Autodesk Fusion 360 part; units mm, degrees
(part 19 of 40)
  line L749 (-24.8392, 62.4581) -> (-24.83, 62.6207) construction
  line L750 (-24.83, 62.6207) -> (-24.8199, 62.7835) construction
  line L751 (-24.8199, 62.7835) -> (-24.8088, 62.9464) construction
  line L752 (-24.8088, 62.9464) -> (-24.7967, 63.1095) construction
  line L753 (-24.7967, 63.1095) -> (-24.7838, 63.2727) construction
  line L754 (-24.7838, 63.2727) -> (-24.77, 63.436) construction
  line L755 (-24.77, 63.436) -> (-24.7552, 63.5995) construction
  line L756 (-24.7552, 63.5995) -> (-24.7396, 63.7631) construction
  line L757 (-24.7396, 63.7631) -> (-24.723, 63.9268) construction
  line L758 (-24.723, 63.9268) -> (-24.7056, 64.0906) construction
  line L759 (-24.7056, 64.0906) -> (-24.6873, 64.2545) construction
  line L760 (-24.6873, 64.2545) -> (-24.6681, 64.4185) construction
  line L761 (-24.6681, 64.4185) -> (-24.648, 64.5826) construction
  line L762 (-24.648, 64.5826) -> (-24.6271, 64.7468) construction
  line L763 (-24.6271, 64.7468) -> (-24.6054, 64.9111) construction
  line L764 (-24.6054, 64.9111) -> (-24.5828, 65.0755) construction
  line L765 (-24.5828, 65.0755) -> (-24.5593, 65.24) construction
  line L766 (-24.5593, 65.24) -> (-24.535, 65.4046) construction
  line L767 (-24.535, 65.4046) -> (-24.5098, 65.5692) construction
  line L768 (-24.5098, 65.5692) -> (-24.4839, 65.734) construction
  line L769 (-24.4839, 65.734) -> (-24.4571, 65.8987) construction
  line L770 (-24.4571, 65.8987) -> (-24.4294, 66.0636) construction
  line L771 (-24.4294, 66.0636) -> (-24.401, 66.2285) construction
  line L772 (-24.401, 66.2285) -> (-24.3718, 66.3935) construction
  line L773 (-24.3718, 66.3935) -> (-24.3417, 66.5585) construction
  line L774 (-24.3417, 66.5585) -> (-24.3108, 66.7236) construction
  line L775 (-24.3108, 66.7236) -> (-24.2792, 66.8887) construction
  line L776 (-24.2792, 66.8887) -> (-24.2532, 67.0208) construction
  line L777 (-24.2532, 67.0208) -> (-24.2334, 67.1199) construction
  line L778 (-24.2334, 67.1199) -> (-24.22, 67.186) construction
  line L779 (-24.22, 67.186) -> (-24.2132, 67.2191) construction
  line L780 (-31.1115, -52.5103) -> (-31.1272, -52.5368) construction
  line L781 (-31.1272, -52.5368) -> (-31.1594, -52.5895) construction
  line L782 (-31.1594, -52.5895) -> (-31.2097, -52.6672) construction
  line L783 (-31.2097, -52.6672) -> (-31.2807, -52.7681) construction
  line L784 (-31.2807, -52.7681) -> (-31.3748, -52.8906) construction
  line L785 (-31.3748, -52.8906) -> (-31.4727, -53.0106) construction
  line L786 (-31.4727, -53.0106) -> (-31.5729, -53.1289) construction
  line L787 (-31.5729, -53.1289) -> (-31.6744, -53.2464) construction
  line L788 (-31.6744, -53.2464) -> (-31.7767, -53.3634) construction
  line L789 (-31.7767, -53.3634) -> (-31.88, -53.4797) construction
  line L790 (-31.88, -53.4797) -> (-31.9844, -53.5951) construction
  line L791 (-31.9844, -53.5951) -> (-32.0903, -53.7094) construction
  line L792 (-32.0903, -53.7094) -> (-32.1981, -53.8224) construction
  line L793 (-32.1981, -53.8224) -> (-32.3077, -53.934) construction
  line L794 (-32.3077, -53.934) -> (-32.419, -54.0444) construction
  line L795 (-32.419, -54.0444) -> (-32.5316, -54.1537) construction
  line L796 (-32.5316, -54.1537) -> (-32.6455, -54.2622) construction
  line L797 (-32.6455, -54.2622) -> (-32.7603, -54.3698) construction
  line L798 (-32.7603, -54.3698) -> (-32.876, -54.4767) construction
  line L799 (-32.876, -54.4767) -> (-32.9927, -54.5828) construction
  line L800 (-32.9927, -54.5828) -> (-33.1105, -54.6881) construction
  line L801 (-33.1105, -54.6881) -> (-33.2292, -54.7926) construction
  line L802 (-33.2292, -54.7926) -> (-33.3491, -54.8961) construction
  line L803 (-33.3491, -54.8961) -> (-33.47, -54.9988) construction
  line L804 (-33.47, -54.9988) -> (-33.5919, -55.1007) construction
  line L805 (-33.5919, -55.1007) -> (-33.7148, -55.2017) construction
  line L806 (-33.7148, -55.2017) -> (-33.8386, -55.302) construction
  line L807 (-33.8386, -55.302) -> (-33.9633, -55.4015) construction
  line L808 (-33.9633, -55.4015) -> (-34.0888, -55.5003) construction
  line L809 (-34.0888, -55.5003) -> (-34.2151, -55.5984) construction
  line L810 (-34.2151, -55.5984) -> (-34.3423, -55.6957) construction
  line L811 (-34.3423, -55.6957) -> (-34.4703, -55.7923) construction
  line L812 (-34.4703, -55.7923) -> (-34.5991, -55.8881) construction
  line L813 (-34.5991, -55.8881) -> (-34.7288, -55.9832) construction
  line L814 (-34.7288, -55.9832) -> (-34.8592, -56.0776) construction
  line L815 (-34.8592, -56.0776) -> (-34.9905, -56.1712) construction
  line L816 (-34.9905, -56.1712) -> (-35.1224, -56.2642) construction
  line L817 (-35.1224, -56.2642) -> (-35.2552, -56.3564) construction
  line L818 (-35.2552, -56.3564) -> (-35.3886, -56.448) construction
  line L819 (-35.3886, -56.448) -> (-35.5228, -56.5388) construction
  line L820 (-35.5228, -56.5388) -> (-35.6577, -56.629) construction
  line L821 (-35.6577, -56.629) -> (-35.7933, -56.7185) construction
  line L822 (-35.7933, -56.7185) -> (-35.9295, -56.8073) construction
  line L823 (-35.9295, -56.8073) -> (-36.0665, -56.8955) construction
  line L824 (-36.0665, -56.8955) -> (-36.2042, -56.9829) construction
  line L825 (-36.2042, -56.9829) -> (-36.3425, -57.0697) construction
  line L826 (-36.3425, -57.0697) -> (-36.4815, -57.1558) construction
  line L827 (-36.4815, -57.1558) -> (-36.6211, -57.2413) construction
  line L828 (-36.6211, -57.2413) -> (-36.7614, -57.3261) construction
  line L829 (-36.7614, -57.3261) -> (-36.9023, -57.4102) construction
  line L830 (-36.9023, -57.4102) -> (-37.0438, -57.4937) construction
  line L831 (-37.0438, -57.4937) -> (-37.186, -57.5765) construction
  line L832 (-37.186, -57.5765) -> (-37.3288, -57.6587) construction
  line L833 (-37.3288, -57.6587) -> (-37.4721, -57.7403) construction
  line L834 (-37.4721, -57.7403) -> (-37.6161, -57.8212) construction
  line L835 (-37.6161, -57.8212) -> (-37.7607, -57.9014) construction
  line L836 (-37.7607, -57.9014) -> (-37.9058, -57.981) construction
  line L837 (-37.9058, -57.981) -> (-38.0515, -58.06) construction
  line L838 (-38.0515, -58.06) -> (-38.1978, -58.1383) construction
  line L839 (-38.1978, -58.1383) -> (-38.3447, -58.216) construction
  line L840 (-38.3447, -58.216) -> (-38.4921, -58.2931) construction
  line L841 (-38.4921, -58.2931) -> (-38.6401, -58.3695) construction
  line L842 (-38.6401, -58.3695) -> (-38.7886, -58.4453) construction
  line L843 (-38.7886, -58.4453) -> (-38.9377, -58.5205) construction
  line L844 (-38.9377, -58.5205) -> (-39.0873, -58.595) construction
  line L845 (-39.0873, -58.595) -> (-39.2374, -58.669) construction
  line L846 (-39.2374, -58.669) -> (-39.3881, -58.7423) construction
  line L847 (-39.3881, -58.7423) -> (-39.5393, -58.8149) construction
  line L848 (-39.5393, -58.8149) -> (-39.6909, -58.887) construction
  line L849 (-39.6909, -58.887) -> (-39.8431, -58.9584) construction
  line L850 (-39.8431, -58.9584) -> (-39.9653, -59.0151) construction
  line L851 (-39.9653, -59.0151) -> (-40.0572, -59.0573) construction
  line L852 (-40.0572, -59.0573) -> (-40.1185, -59.0853) construction
  line L853 (-40.1185, -59.0853) -> (-40.1492, -59.0993) construction
  line L854 (-52.5103, 31.1115) -> (-52.5368, 31.1272) construction
  line L855 (-52.5368, 31.1272) -> (-52.5895, 31.1594) construction
  line L856 (-52.5895, 31.1594) -> (-52.6672, 31.2097) construction
  line L857 (-52.6672, 31.2097) -> (-52.7681, 31.2807) construction
  line L858 (-52.7681, 31.2807) -> (-52.8906, 31.3748) construction
  line L859 (-52.8906, 31.3748) -> (-53.0106, 31.4727) construction
  line L860 (-53.0106, 31.4727) -> (-53.1289, 31.5729) construction
  line L861 (-53.1289, 31.5729) -> (-53.2464, 31.6744) construction
  line L862 (-53.2464, 31.6744) -> (-53.3634, 31.7767) construction
  line L863 (-53.3634, 31.7767) -> (-53.4797, 31.88) construction
  line L864 (-53.4797, 31.88) -> (-53.5951, 31.9844) construction
  line L865 (-53.5951, 31.9844) -> (-53.7094, 32.0903) construction
  line L866 (-53.7094, 32.0903) -> (-53.8224, 32.1981) construction
  line L867 (-53.8224, 32.1981) -> (-53.934, 32.3077) construction
  line L868 (-53.934, 32.3077) -> (-54.0444, 32.419) construction
  line L869 (-54.0444, 32.419) -> (-54.1537, 32.5316) construction
  line L870 (-54.1537, 32.5316) -> (-54.2622, 32.6455) construction
  line L871 (-54.2622, 32.6455) -> (-54.3698, 32.7603) construction
  line L872 (-54.3698, 32.7603) -> (-54.4767, 32.876) construction
  line L873 (-54.4767, 32.876) -> (-54.5828, 32.9927) construction
  line L874 (-54.5828, 32.9927) -> (-54.6881, 33.1105) construction
  line L875 (-54.6881, 33.1105) -> (-54.7926, 33.2292) construction
  line L876 (-54.7926, 33.2292) -> (-54.8961, 33.3491) construction
  line L877 (-54.8961, 33.3491) -> (-54.9988, 33.47) construction
  line L878 (-54.9988, 33.47) -> (-55.1007, 33.5919) construction
  line L879 (-55.1007, 33.5919) -> (-55.2017, 33.7148) construction
  line L880 (-55.2017, 33.7148) -> (-55.302, 33.8386) construction
  line L881 (-55.302, 33.8386) -> (-55.4015, 33.9633) construction
  line L882 (-55.4015, 33.9633) -> (-55.5003, 34.0888) construction
  line L883 (-55.5003, 34.0888) -> (-55.5984, 34.2151) construction
  line L884 (-55.5984, 34.2151) -> (-55.6957, 34.3423) construction
  line L885 (-55.6957, 34.3423) -> (-55.7923, 34.4703) construction
  line L886 (-55.7923, 34.4703) -> (-55.8881, 34.5991) construction
  line L887 (-55.8881, 34.5991) -> (-55.9832, 34.7288) construction
  line L888 (-55.9832, 34.7288) -> (-56.0776, 34.8592) construction
  line L889 (-56.0776, 34.8592) -> (-56.1712, 34.9905) construction
  line L890 (-56.1712, 34.9905) -> (-56.2642, 35.1224) construction
  line L891 (-56.2642, 35.1224) -> (-56.3564, 35.2552) construction
  line L892 (-56.3564, 35.2552) -> (-56.448, 35.3886) construction
  line L893 (-56.448, 35.3886) -> (-56.5388, 35.5228) construction
  line L894 (-56.5388, 35.5228) -> (-56.629, 35.6577) construction
  line L895 (-56.629, 35.6577) -> (-56.7185, 35.7933) construction
  line L896 (-56.7185, 35.7933) -> (-56.8073, 35.9295) construction
  line L897 (-56.8073, 35.9295) -> (-56.8955, 36.0665) construction
  line L898 (-56.8955, 36.0665) -> (-56.9829, 36.2042) construction
  line L899 (-56.9829, 36.2042) -> (-57.0697, 36.3425) construction
  line L900 (-57.0697, 36.3425) -> (-57.1558, 36.4815) construction
  line L901 (-57.1558, 36.4815) -> (-57.2413, 36.6211) construction
  line L902 (-57.2413, 36.6211) -> (-57.3261, 36.7614) construction
  line L903 (-57.3261, 36.7614) -> (-57.4102, 36.9023) construction
  line L904 (-57.4102, 36.9023) -> (-57.4937, 37.0438) construction
  line L905 (-57.4937, 37.0438) -> (-57.5765, 37.186) construction
  line L906 (-57.5765, 37.186) -> (-57.6587, 37.3288) construction
  line L907 (-57.6587, 37.3288) -> (-57.7403, 37.4721) construction
  line L908 (-57.7403, 37.4721) -> (-57.8212, 37.6161) construction
  line L909 (-57.8212, 37.6161) -> (-57.9014, 37.7607) construction
  line L910 (-57.9014, 37.7607) -> (-57.981, 37.9058) construction
  line L911 (-57.981, 37.9058) -> (-58.06, 38.0515) construction
  line L912 (-58.06, 38.0515) -> (-58.1383, 38.1978) construction
  line L913 (-58.1383, 38.1978) -> (-58.216, 38.3447) construction
  line L914 (-58.216, 38.3447) -> (-58.2931, 38.4921) construction
  line L915 (-58.2931, 38.4921) -> (-58.3695, 38.6401) construction
  line L916 (-58.3695, 38.6401) -> (-58.4453, 38.7886) construction
  line L917 (-58.4453, 38.7886) -> (-58.5205, 38.9377) construction
  line L918 (-58.5205, 38.9377) -> (-58.595, 39.0873) construction
  line L919 (-58.595, 39.0873) -> (-58.669, 39.2374) construction
  line L920 (-58.669, 39.2374) -> (-58.7423, 39.3881) construction
  line L921 (-58.7423, 39.3881) -> (-58.8149, 39.5393) construction
  line L922 (-58.8149, 39.5393) -> (-58.887, 39.6909) construction
  line L923 (-58.887, 39.6909) -> (-58.9584, 39.8431) construction
  line L924 (-58.9584, 39.8431) -> (-59.0151, 39.9653) construction
  line L925 (-59.0151, 39.9653) -> (-59.0573, 40.0572) construction
  line L926 (-59.0573, 40.0572) -> (-59.0853, 40.1185) construction
  line L927 (-59.0853, 40.1185) -> (-59.0993, 40.1492) construction
  line L928 (5.6951, 60.7685) -> (5.6979, 60.7993) construction
  line L929 (5.6979, 60.7993) -> (5.7029, 60.8609) construction
  line L930 (5.7029, 60.8609) -> (5.7078, 60.9533) construction
  line L931 (5.7078, 60.9533) -> (5.7097, 61.0766) construction
  line L932 (5.7097, 61.0766) -> (5.7056, 61.231) construction
  line L933 (5.7056, 61.231) -> (5.6969, 61.3856) construction
  line L934 (5.6969, 61.3856) -> (5.6854, 61.5403) construction
  line L935 (5.6854, 61.5403) -> (5.6723, 61.695) construction
  line L936 (5.6723, 61.695) -> (5.6583, 61.8498) construction
  line L937 (5.6583, 61.8498) -> (5.6431, 62.0045) construction
  line L938 (5.6431, 62.0045) -> (5.6265, 62.1593) construction
  line L939 (5.6265, 62.1593) -> (5.608, 62.314) construction
  line L940 (5.608, 62.314) -> (5.5871, 62.4688) construction
  line L941 (5.5871, 62.4688) -> (5.5641, 62.6235) construction
  line L942 (5.5641, 62.6235) -> (5.539, 62.7782) construction
  line L943 (5.539, 62.7782) -> (5.5121, 62.9329) construction
  line L944 (5.5121, 62.9329) -> (5.4838, 63.0875) construction
  line L945 (5.4838, 63.0875) -> (5.4542, 63.2421) construction
  line L946 (5.4542, 63.2421) -> (5.4233, 63.3966) construction
  line L947 (5.4233, 63.3966) -> (5.3913, 63.5511) construction
  line L948 (5.3913, 63.5511) -> (5.3579, 63.7055) construction
  line L949 (5.3579, 63.7055) -> (5.3232, 63.8598) construction
  line L950 (5.3232, 63.8598) -> (5.2871, 64.014) construction
  line L951 (5.2871, 64.014) -> (5.2497, 64.1682) construction
  line L952 (5.2497, 64.1682) -> (5.2109, 64.3222) construction
  line L953 (5.2109, 64.3222) -> (5.1709, 64.4762) construction
  line L954 (5.1709, 64.4762) -> (5.1297, 64.6301) construction
  line L955 (5.1297, 64.6301) -> (5.0873, 64.7839) construction
  line L956 (5.0873, 64.7839) -> (5.0439, 64.9376) construction
  line L957 (5.0439, 64.9376) -> (4.9993, 65.0912) construction
  line L958 (4.9993, 65.0912) -> (4.9536, 65.2447) construction
  line L959 (4.9536, 65.2447) -> (4.9068, 65.398) construction
  line L960 (4.9068, 65.398) -> (4.8589, 65.5513) construction
  line L961 (4.8589, 65.5513) -> (4.8099, 65.7044) construction
  line L962 (4.8099, 65.7044) -> (4.7599, 65.8574) construction
  line L963 (4.7599, 65.8574) -> (4.7087, 66.0103) construction
  line L964 (4.7087, 66.0103) -> (4.6566, 66.1631) construction
  line L965 (4.6566, 66.1631) -> (4.6035, 66.3158) construction
  line L966 (4.6035, 66.3158) -> (4.5493, 66.4683) construction
  line L967 (4.5493, 66.4683) -> (4.4942, 66.6206) construction
  line L968 (4.4942, 66.6206) -> (4.438, 66.7729) construction
  line L969 (4.438, 66.7729) -> (4.381, 66.925) construction
  line L970 (4.381, 66.925) -> (4.3229, 67.077) construction
  line L971 (4.3229, 67.077) -> (4.2639, 67.2288) construction
  line L972 (4.2639, 67.2288) -> (4.2039, 67.3804) construction
  line L973 (4.2039, 67.3804) -> (4.143, 67.532) construction
  line L974 (4.143, 67.532) -> (4.0812, 67.6833) construction
  line L975 (4.0812, 67.6833) -> (4.0185, 67.8345) construction
  line L976 (4.0185, 67.8345) -> (3.9548, 67.9856) construction
  line L977 (3.9548, 67.9856) -> (3.8903, 68.1365) construction
  line L978 (3.8903, 68.1365) -> (3.8249, 68.2872) construction
  line L979 (3.8249, 68.2872) -> (3.7585, 68.4378) construction
  line L980 (3.7585, 68.4378) -> (3.6913, 68.5882) construction
  line L981 (3.6913, 68.5882) -> (3.6233, 68.7384) construction
  line L982 (3.6233, 68.7384) -> (3.5543, 68.8885) construction
  line L983 (3.5543, 68.8885) -> (3.4846, 69.0384) construction
  line L984 (3.4846, 69.0384) -> (3.4139, 69.1881) construction
  line L985 (3.4139, 69.1881) -> (3.3425, 69.3376) construction
  line L986 (3.3425, 69.3376) -> (3.2701, 69.487) construction
  line L987 (3.2701, 69.487) -> (3.197, 69.6362) construction
  line L988 (3.197, 69.6362) -> (3.123, 69.7852) construction
  line L989 (3.123, 69.7852) -> (3.0482, 69.934) construction
  line L990 (3.0482, 69.934) -> (2.9726, 70.0826) construction
  line L991 (2.9726, 70.0826) -> (2.8962, 70.2311) construction
  line L992 (2.8962, 70.2311) -> (2.819, 70.3793) construction
  line L993 (2.819, 70.3793) -> (2.741, 70.5274) construction
  line L994 (2.741, 70.5274) -> (2.6622, 70.6752) construction
  line L995 (2.6622, 70.6752) -> (2.5826, 70.8229) construction
  line L996 (2.5826, 70.8229) -> (2.5023, 70.9703) construction
  line L997 (2.5023, 70.9703) -> (2.4211, 71.1176) construction
  line L998 (2.4211, 71.1176) -> (2.3556, 71.2352) construction
  line L999 (2.3556, 71.2352) -> (2.3061, 71.3234) construction
  line L1000 (2.3061, 71.3234) -> (2.2729, 71.3821) construction
  line L1001 (2.2729, 71.3821) -> (2.2563, 71.4115) construction
  line L1002 (40.3263, 45.8153) -> (40.3467, 45.8385) construction
  line L1003 (40.3467, 45.8385) -> (40.3868, 45.8854) construction
  line L1004 (40.3868, 45.8854) -> (40.4451, 45.9573) construction
  line L1005 (40.4451, 45.9573) -> (40.5192, 46.056) construction
  line L1006 (40.5192, 46.056) -> (40.6066, 46.1833) construction
  line L1007 (40.6066, 46.1833) -> (40.6904, 46.3135) construction
  line L1008 (40.6904, 46.3135) -> (40.772, 46.4454) construction
  line L1009 (40.772, 46.4454) -> (40.8524, 46.5782) construction
  line L1010 (40.8524, 46.5782) -> (40.932, 46.7117) construction
  line L1011 (40.932, 46.7117) -> (41.0107, 46.8458) construction
  line L1012 (41.0107, 46.8458) -> (41.0883, 46.9807) construction
  line L1013 (41.0883, 46.9807) -> (41.1642, 47.1168) construction
  line L1014 (41.1642, 47.1168) -> (41.2383, 47.2543) construction
  line L1015 (41.2383, 47.2543) -> (41.3106, 47.393) construction
  line L1016 (41.3106, 47.393) -> (41.3813, 47.5329) construction
  line L1017 (41.3813, 47.5329) -> (41.4504, 47.6738) construction
  line L1018 (41.4504, 47.6738) -> (41.5184, 47.8156) construction
  line L1019 (41.5184, 47.8156) -> (41.5853, 47.9581) construction
  line L1020 (41.5853, 47.9581) -> (41.6512, 48.1012) construction
  line L1021 (41.6512, 48.1012) -> (41.716, 48.245) construction
  line L1022 (41.716, 48.245) -> (41.7798, 48.3895) construction
  line L1023 (41.7798, 48.3895) -> (41.8424, 48.5347) construction
  line L1024 (41.8424, 48.5347) -> (41.9039, 48.6807) construction
  line L1025 (41.9039, 48.6807) -> (41.9642, 48.8274) construction
  line L1026 (41.9642, 48.8274) -> (42.0234, 48.9749) construction
  line L1027 (42.0234, 48.9749) -> (42.0815, 49.123) construction
  line L1028 (42.0815, 49.123) -> (42.1386, 49.2717) construction
  line L1029 (42.1386, 49.2717) -> (42.1947, 49.421) construction
  line L1030 (42.1947, 49.421) -> (42.2499, 49.5709) construction
  line L1031 (42.2499, 49.5709) -> (42.3041, 49.7214) construction
  line L1032 (42.3041, 49.7214) -> (42.3574, 49.8724) construction
  line L1033 (42.3574, 49.8724) -> (42.4097, 50.024) construction
  line L1034 (42.4097, 50.024) -> (42.461, 50.1761) construction
  line L1035 (42.461, 50.1761) -> (42.5114, 50.3288) construction
  line L1036 (42.5114, 50.3288) -> (42.5608, 50.482) construction
  line L1037 (42.5608, 50.482) -> (42.6094, 50.6358) construction
  line L1038 (42.6094, 50.6358) -> (42.657, 50.79) construction
  line L1039 (42.657, 50.79) -> (42.7037, 50.9447) construction
  line L1040 (42.7037, 50.9447) -> (42.7495, 51.0999) construction
  line L1041 (42.7495, 51.0999) -> (42.7945, 51.2556) construction
  line L1042 (42.7945, 51.2556) -> (42.8386, 51.4118) construction
  line L1043 (42.8386, 51.4118) -> (42.8818, 51.5684) construction
  line L1044 (42.8818, 51.5684) -> (42.9241, 51.7255) construction
  line L1045 (42.9241, 51.7255) -> (42.9656, 51.883) construction
  line L1046 (42.9656, 51.883) -> (43.0063, 52.0409) construction
  line L1047 (43.0063, 52.0409) -> (43.0461, 52.1993) construction
  line L1048 (43.0461, 52.1993) -> (43.085, 52.3581) construction
  line L1049 (43.085, 52.3581) -> (43.1231, 52.5173) construction
  line L1050 (43.1231, 52.5173) -> (43.1604, 52.6769) construction
  line L1051 (43.1604, 52.6769) -> (43.1969, 52.8369) construction
  line L1052 (43.1969, 52.8369) -> (43.2326, 52.9973) construction
  line L1053 (43.2326, 52.9973) -> (43.2674, 53.1581) construction
  line L1054 (43.2674, 53.1581) -> (43.3015, 53.3193) construction
  line L1055 (43.3015, 53.3193) -> (43.3347, 53.4809) construction
  line L1056 (43.3347, 53.4809) -> (43.3672, 53.6428) construction
  line L1057 (43.3672, 53.6428) -> (43.3988, 53.8051) construction
  line L1058 (43.3988, 53.8051) -> (43.4297, 53.9677) construction
  line L1059 (43.4297, 53.9677) -> (43.4597, 54.1307) construction
  line L1060 (43.4597, 54.1307) -> (43.489, 54.294) construction
  line L1061 (43.489, 54.294) -> (43.5175, 54.4577) construction
  line L1062 (43.5175, 54.4577) -> (43.5453, 54.6217) construction
  line L1063 (43.5453, 54.6217) -> (43.5723, 54.7861) construction
  line L1064 (43.5723, 54.7861) -> (43.5984, 54.9508) construction
  line L1065 (43.5984, 54.9508) -> (43.6239, 55.1158) construction
  line L1066 (43.6239, 55.1158) -> (43.6486, 55.2811) construction
  line L1067 (43.6486, 55.2811) -> (43.6725, 55.4467) construction
  line L1068 (43.6725, 55.4467) -> (43.6956, 55.6126) construction
  line L1069 (43.6956, 55.6126) -> (43.718, 55.7789) construction
  line L1070 (43.718, 55.7789) -> (43.7397, 55.9454) construction
  line L1071 (43.7397, 55.9454) -> (43.7606, 56.1122) construction
  line L1072 (43.7606, 56.1122) -> (43.7767, 56.2459) construction
  line L1073 (43.7767, 56.2459) -> (43.7885, 56.3463) construction
  line L1074 (43.7885, 56.3463) -> (43.7962, 56.4133) construction
  line L1075 (43.7962, 56.4133) -> (43.8, 56.4469) construction
  line L1076 (-59.5542, -13.3622) -> (-59.5843, -13.369) construction
  line L1077 (-59.5843, -13.369) -> (-59.6444, -13.3833) construction
  line L1078 (-59.6444, -13.3833) -> (-59.7338, -13.4071) construction
  line L1079 (-59.7338, -13.4071) -> (-59.8517, -13.4435) construction
  line L1080 (-59.8517, -13.4435) -> (-59.9973, -13.4951) construction
  line L1081 (-59.9973, -13.4951) -> (-60.1416, -13.5511) construction
  line L1082 (-60.1416, -13.5511) -> (-60.2852, -13.6099) construction
  line L1083 (-60.2852, -13.6099) -> (-60.4283, -13.6701) construction
  line L1084 (-60.4283, -13.6701) -> (-60.5711, -13.7313) construction
  line L1085 (-60.5711, -13.7313) -> (-60.7136, -13.7935) construction
  line L1086 (-60.7136, -13.7935) -> (-60.8557, -13.8571) construction
  line L1087 (-60.8557, -13.8571) -> (-60.9971, -13.9226) construction
  line L1088 (-60.9971, -13.9226) -> (-61.1379, -13.9902) construction
  line L1089 (-61.1379, -13.9902) -> (-61.2779, -14.06) construction
  line L1090 (-61.2779, -14.06) -> (-61.4173, -14.1316) construction
  line L1091 (-61.4173, -14.1316) -> (-61.5561, -14.205) construction
  line L1092 (-61.5561, -14.205) -> (-61.6944, -14.2797) construction
  line L1093 (-61.6944, -14.2797) -> (-61.8322, -14.3557) construction
  line L1094 (-61.8322, -14.3557) -> (-61.9697, -14.4327) construction
  line L1095 (-61.9697, -14.4327) -> (-62.1067, -14.5109) construction
  line L1096 (-62.1067, -14.5109) -> (-62.2432, -14.5904) construction
  line L1097 (-62.2432, -14.5904) -> (-62.3792, -14.6711) construction
  line L1098 (-62.3792, -14.6711) -> (-62.5148, -14.753) construction
  line L1099 (-62.5148, -14.753) -> (-62.6498, -14.8363) construction
  line L1100 (-62.6498, -14.8363) -> (-62.7843, -14.9208) construction
  line L1101 (-62.7843, -14.9208) -> (-62.9184, -15.0064) construction
  line L1102 (-62.9184, -15.0064) -> (-63.052, -15.0932) construction
  line L1103 (-63.052, -15.0932) -> (-63.1852, -15.181) construction
  line L1104 (-63.1852, -15.181) -> (-63.318, -15.2698) construction
  line L1105 (-63.318, -15.2698) -> (-63.4503, -15.3597) construction
  line L1106 (-63.4503, -15.3597) -> (-63.5821, -15.4506) construction
  line L1107 (-63.5821, -15.4506) -> (-63.7135, -15.5425) construction
  line L1108 (-63.7135, -15.5425) -> (-63.8445, -15.6354) construction
  line L1109 (-63.8445, -15.6354) -> (-63.975, -15.7293) construction
  line L1110 (-63.975, -15.7293) -> (-64.105, -15.8242) construction
  line L1111 (-64.105, -15.8242) -> (-64.2346, -15.92) construction
  line L1112 (-64.2346, -15.92) -> (-64.3638, -16.0168) construction
  line L1113 (-64.3638, -16.0168) -> (-64.4926, -16.1146) construction
  line L1114 (-64.4926, -16.1146) -> (-64.6209, -16.2132) construction
  line L1115 (-64.6209, -16.2132) -> (-64.7488, -16.3127) construction
  line L1116 (-64.7488, -16.3127) -> (-64.8762, -16.4131) construction
  line L1117 (-64.8762, -16.4131) -> (-65.0032, -16.5144) construction
  line L1118 (-65.0032, -16.5144) -> (-65.1298, -16.6166) construction
  line L1119 (-65.1298, -16.6166) -> (-65.256, -16.7196) construction
  line L1120 (-65.256, -16.7196) -> (-65.3817, -16.8235) construction
  line L1121 (-65.3817, -16.8235) -> (-65.507, -16.9283) construction
  line L1122 (-65.507, -16.9283) -> (-65.6318, -17.0338) construction
  line L1123 (-65.6318, -17.0338) -> (-65.7562, -17.1402) construction
  line L1124 (-65.7562, -17.1402) -> (-65.8802, -17.2474) construction
  line L1125 (-65.8802, -17.2474) -> (-66.0038, -17.3555) construction
  line L1126 (-66.0038, -17.3555) -> (-66.1269, -17.4643) construction
  line L1127 (-66.1269, -17.4643) -> (-66.2497, -17.5739) construction
  line L1128 (-66.2497, -17.5739) -> (-66.3719, -17.6842) construction
  line L1129 (-66.3719, -17.6842) -> (-66.4938, -17.7954) construction
  line L1130 (-66.4938, -17.7954) -> (-66.6152, -17.9073) construction
  line L1131 (-66.6152, -17.9073) -> (-66.7362, -18.02) construction
  line L1132 (-66.7362, -18.02) -> (-66.8568, -18.1335) construction
  line L1133 (-66.8568, -18.1335) -> (-66.9769, -18.2477) construction
  line L1134 (-66.9769, -18.2477) -> (-67.0966, -18.3626) construction
  line L1135 (-67.0966, -18.3626) -> (-67.2159, -18.4782) construction
  line L1136 (-67.2159, -18.4782) -> (-67.3347, -18.5946) construction
  line L1137 (-67.3347, -18.5946) -> (-67.4531, -18.7118) construction
  line L1138 (-67.4531, -18.7118) -> (-67.5711, -18.8296) construction
  line L1139 (-67.5711, -18.8296) -> (-67.6887, -18.9481) construction
  line L1140 (-67.6887, -18.9481) -> (-67.8058, -19.0674) construction
  line L1141 (-67.8058, -19.0674) -> (-67.9225, -19.1873) construction
  line L1142 (-67.9225, -19.1873) -> (-68.0388, -19.3079) construction
  line L1143 (-68.0388, -19.3079) -> (-68.1546, -19.4293) construction
  line L1144 (-68.1546, -19.4293) -> (-68.27, -19.5512) construction
  line L1145 (-68.27, -19.5512) -> (-68.385, -19.6739) construction
  line L1146 (-68.385, -19.6739) -> (-68.4767, -19.7726) construction
  line L1147 (-68.4767, -19.7726) -> (-68.5452, -19.8469) construction
  line L1148 (-68.5452, -19.8469) -> (-68.5908, -19.8966) construction
  line L1149 (-68.5908, -19.8966) -> (-68.6136, -19.9215) construction
  line L1150 (-52.5103, -31.1115) -> (-52.5368, -31.1272) construction
  line L1151 (-52.5368, -31.1272) -> (-52.5895, -31.1594) construction
  line L1152 (-52.5895, -31.1594) -> (-52.6672, -31.2097) construction
  line L1153 (-52.6672, -31.2097) -> (-52.7681, -31.2807) construction
  line L1154 (-52.7681, -31.2807) -> (-52.8906, -31.3748) construction
  line L1155 (-52.8906, -31.3748) -> (-53.0106, -31.4727) construction
  line L1156 (-53.0106, -31.4727) -> (-53.1289, -31.5729) construction
  line L1157 (-53.1289, -31.5729) -> (-53.2464, -31.6744) construction
  line L1158 (-53.2464, -31.6744) -> (-53.3634, -31.7767) construction
  line L1159 (-53.3634, -31.7767) -> (-53.4797, -31.88) construction
  line L1160 (-53.4797, -31.88) -> (-53.5951, -31.9844) construction
  line L1161 (-53.5951, -31.9844) -> (-53.7094, -32.0903) construction
  line L1162 (-53.7094, -32.0903) -> (-53.8224, -32.1981) construction
  line L1163 (-53.8224, -32.1981) -> (-53.934, -32.3077) construction
  line L1164 (-53.934, -32.3077) -> (-54.0444, -32.419) construction
  line L1165 (-54.0444, -32.419) -> (-54.1537, -32.5316) construction
  line L1166 (-54.1537, -32.5316) -> (-54.2622, -32.6455) construction
  line L1167 (-54.2622, -32.6455) -> (-54.3698, -32.7603) construction
  line L1168 (-54.3698, -32.7603) -> (-54.4767, -32.876) construction
  line L1169 (-54.4767, -32.876) -> (-54.5828, -32.9927) construction
  line L1170 (-54.5828, -32.9927) -> (-54.6881, -33.1105) construction
  line L1171 (-54.6881, -33.1105) -> (-54.7926, -33.2292) construction
  line L1172 (-54.7926, -33.2292) -> (-54.8961, -33.3491) construction
  line L1173 (-54.8961, -33.3491) -> (-54.9988, -33.47) construction
  line L1174 (-54.9988, -33.47) -> (-55.1007, -33.5919) construction
  line L1175 (-55.1007, -33.5919) -> (-55.2017, -33.7148) construction
  line L1176 (-55.2017, -33.7148) -> (-55.302, -33.8386) construction
  line L1177 (-55.302, -33.8386) -> (-55.4015, -33.9633) construction
  line L1178 (-55.4015, -33.9633) -> (-55.5003, -34.0888) construction
  line L1179 (-55.5003, -34.0888) -> (-55.5984, -34.2151) construction
  line L1180 (-55.5984, -34.2151) -> (-55.6957, -34.3423) construction
  line L1181 (-55.6957, -34.3423) -> (-55.7923, -34.4703) construction
  line L1182 (-55.7923, -34.4703) -> (-55.8881, -34.5991) construction
  line L1183 (-55.8881, -34.5991) -> (-55.9832, -34.7288) construction
  line L1184 (-55.9832, -34.7288) -> (-56.0776, -34.8592) construction
  line L1185 (-56.0776, -34.8592) -> (-56.1712, -34.9905) construction
  line L1186 (-56.1712, -34.9905) -> (-56.2642, -35.1224) construction
  line L1187 (-56.2642, -35.1224) -> (-56.3564, -35.2552) construction
  line L1188 (-56.3564, -35.2552) -> (-56.448, -35.3886) construction
  line L1189 (-56.448, -35.3886) -> (-56.5388, -35.5228) construction
  line L1190 (-56.5388, -35.5228) -> (-56.629, -35.6577) construction
  line L1191 (-56.629, -35.6577) -> (-56.7185, -35.7933) construction
  line L1192 (-56.7185, -35.7933) -> (-56.8073, -35.9295) construction
  line L1193 (-56.8073, -35.9295) -> (-56.8955, -36.0665) construction
  line L1194 (-56.8955, -36.0665) -> (-56.9829, -36.2042) construction
  line L1195 (-56.9829, -36.2042) -> (-57.0697, -36.3425) construction
  line L1196 (-57.0697, -36.3425) -> (-57.1558, -36.4815) construction
  line L1197 (-57.1558, -36.4815) -> (-57.2413, -36.6211) construction
  line L1198 (-57.2413, -36.6211) -> (-57.3261, -36.7614) construction
  line L1199 (-57.3261, -36.7614) -> (-57.4102, -36.9023) construction
  line L1200 (-57.4102, -36.9023) -> (-57.4937, -37.0438) construction
  line L1201 (-57.4937, -37.0438) -> (-57.5765, -37.186) construction
  line L1202 (-57.5765, -37.186) -> (-57.6587, -37.3288) construction
  line L1203 (-57.6587, -37.3288) -> (-57.7403, -37.4721) construction
  line L1204 (-57.7403, -37.4721) -> (-57.8212, -37.6161) construction
  line L1205 (-57.8212, -37.6161) -> (-57.9014, -37.7607) construction
  line L1206 (-57.9014, -37.7607) -> (-57.981, -37.9058) construction
  line L1207 (-57.981, -37.9058) -> (-58.06, -38.0515) construction
  line L1208 (-58.06, -38.0515) -> (-58.1383, -38.1978) construction
  line L1209 (-58.1383, -38.1978) -> (-58.216, -38.3447) construction
  line L1210 (-58.216, -38.3447) -> (-58.2931, -38.4921) construction
  line L1211 (-58.2931, -38.4921) -> (-58.3695, -38.6401) construction
  line L1212 (-58.3695, -38.6401) -> (-58.4453, -38.7886) construction
  line L1213 (-58.4453, -38.7886) -> (-58.5205, -38.9377) construction
  line L1214 (-58.5205, -38.9377) -> (-58.595, -39.0873) construction
  line L1215 (-58.595, -39.0873) -> (-58.669, -39.2374) construction
  line L1216 (-58.669, -39.2374) -> (-58.7423, -39.3881) construction
  line L1217 (-58.7423, -39.3881) -> (-58.8149, -39.5393) construction
  line L1218 (-58.8149, -39.5393) -> (-58.887, -39.6909) construction
  line L1219 (-58.887, -39.6909) -> (-58.9584, -39.8431) construction
  line L1220 (-58.9584, -39.8431) -> (-59.0151, -39.9653) construction
  line L1221 (-59.0151, -39.9653) -> (-59.0573, -40.0572) construction
  line L1222 (-59.0573, -40.0572) -> (-59.0853, -40.1185) construction
  line L1223 (-59.0853, -40.1185) -> (-59.0993, -40.1492) construction
  line L1224 (-56.0345, -24.1948) -> (-56.0628, -24.2071) construction
  line L1225 (-56.0628, -24.2071) -> (-56.1198, -24.2308) construction
  line L1226 (-56.1198, -24.2308) -> (-56.2062, -24.264) construction
  line L1227 (-56.2062, -24.264) -> (-56.3229, -24.3039) construction
  line L1228 (-56.3229, -24.3039) -> (-56.4711, -24.3478) construction
  line L1229 (-56.4711, -24.3478) -> (-56.6208, -24.3873) construction
  line L1230 (-56.6208, -24.3873) -> (-56.7714, -24.4241) construction
  line L1231 (-56.7714, -24.4241) -> (-56.9226, -24.4595) construction
  line L1232 (-56.9226, -24.4595) -> (-57.0741, -24.494) construction
  line L1233 (-57.0741, -24.494) -> (-57.226, -24.5274) construction
  line L1234 (-57.226, -24.5274) -> (-57.3783, -24.5594) construction
  line L1235 (-57.3783, -24.5594) -> (-57.5312, -24.5896) construction
  line L1236 (-57.5312, -24.5896) -> (-57.6848, -24.6176) construction
  line L1237 (-57.6848, -24.6176) -> (-57.8391, -24.6435) construction
  line L1238 (-57.8391, -24.6435) -> (-57.994, -24.6674) construction
  line L1239 (-57.994, -24.6674) -> (-58.1494, -24.6897) construction
  line L1240 (-58.1494, -24.6897) -> (-58.3052, -24.7105) construction
  line L1241 (-58.3052, -24.7105) -> (-58.4614, -24.7301) construction
  line L1242 (-58.4614, -24.7301) -> (-58.6179, -24.7485) construction
  line L1243 (-58.6179, -24.7485) -> (-58.7747, -24.7658) construction
  line L1244 (-58.7747, -24.7658) -> (-58.9318, -24.7818) construction
  line L1245 (-58.9318, -24.7818) -> (-59.0893, -24.7965) construction
  line L1246 (-59.0893, -24.7965) -> (-59.2471, -24.8098) construction
  line L1247 (-59.2471, -24.8098) -> (-59.4053, -24.8218) construction
  line L1248 (-59.4053, -24.8218) -> (-59.5638, -24.8325) construction
  line L1249 (-59.5638, -24.8325) -> (-59.7226, -24.842) construction
  line L1250 (-59.7226, -24.842) -> (-59.8817, -24.8504) construction
  line L1251 (-59.8817, -24.8504) -> (-60.0411, -24.8577) construction
  line L1252 (-60.0411, -24.8577) -> (-60.2007, -24.8638) construction
  line L1253 (-60.2007, -24.8638) -> (-60.3605, -24.8689) construction
  line L1254 (-60.3605, -24.8689) -> (-60.5206, -24.8729) construction
  line L1255 (-60.5206, -24.8729) -> (-60.6809, -24.8757) construction
  line L1256 (-60.6809, -24.8757) -> (-60.8415, -24.8776) construction
  line L1257 (-60.8415, -24.8776) -> (-61.0023, -24.8783) construction
  line L1258 (-61.0023, -24.8783) -> (-61.1633, -24.878) construction
  line L1259 (-61.1633, -24.878) -> (-61.3245, -24.8766) construction
  line L1260 (-61.3245, -24.8766) -> (-61.4859, -24.8742) construction
  line L1261 (-61.4859, -24.8742) -> (-61.6475, -24.8708) construction
  line L1262 (-61.6475, -24.8708) -> (-61.8093, -24.8665) construction
  line L1263 (-61.8093, -24.8665) -> (-61.9712, -24.8611) construction
  line L1264 (-61.9712, -24.8611) -> (-62.1334, -24.8548) construction
  line L1265 (-62.1334, -24.8548) -> (-62.2957, -24.8475) construction
  line L1266 (-62.2957, -24.8475) -> (-62.4581, -24.8392) construction
  line L1267 (-62.4581, -24.8392) -> (-62.6207, -24.83) construction
  line L1268 (-62.6207, -24.83) -> (-62.7835, -24.8199) construction
  line L1269 (-62.7835, -24.8199) -> (-62.9464, -24.8088) construction
  line L1270 (-62.9464, -24.8088) -> (-63.1095, -24.7967) construction
  line L1271 (-63.1095, -24.7967) -> (-63.2727, -24.7838) construction
  line L1272 (-63.2727, -24.7838) -> (-63.436, -24.77) construction
  line L1273 (-63.436, -24.77) -> (-63.5995, -24.7552) construction
  line L1274 (-63.5995, -24.7552) -> (-63.7631, -24.7396) construction
  line L1275 (-63.7631, -24.7396) -> (-63.9268, -24.723) construction
  line L1276 (-63.9268, -24.723) -> (-64.0906, -24.7056) construction
  line L1277 (-64.0906, -24.7056) -> (-64.2545, -24.6873) construction
  line L1278 (-64.2545, -24.6873) -> (-64.4185, -24.6681) construction
  line L1279 (-64.4185, -24.6681) -> (-64.5826, -24.648) construction
  line L1280 (-64.5826, -24.648) -> (-64.7468, -24.6271) construction
  line L1281 (-64.7468, -24.6271) -> (-64.9111, -24.6054) construction
  line L1282 (-64.9111, -24.6054) -> (-65.0755, -24.5828) construction
  line L1283 (-65.0755, -24.5828) -> (-65.24, -24.5593) construction
  line L1284 (-65.24, -24.5593) -> (-65.4046, -24.535) construction
  line L1285 (-65.4046, -24.535) -> (-65.5692, -24.5098) construction
  line L1286 (-65.5692, -24.5098) -> (-65.734, -24.4839) construction
  line L1287 (-65.734, -24.4839) -> (-65.8987, -24.4571) construction
  line L1288 (-65.8987, -24.4571) -> (-66.0636, -24.4294) construction
  line L1289 (-66.0636, -24.4294) -> (-66.2285, -24.401) construction
  line L1290 (-66.2285, -24.401) -> (-66.3935, -24.3718) construction
  line L1291 (-66.3935, -24.3718) -> (-66.5585, -24.3417) construction
  line L1292 (-66.5585, -24.3417) -> (-66.7236, -24.3108) construction
  line L1293 (-66.7236, -24.3108) -> (-66.8887, -24.2792) construction
  line L1294 (-66.8887, -24.2792) -> (-67.0208, -24.2532) construction
  line L1295 (-67.0208, -24.2532) -> (-67.1199, -24.2334) construction
  line L1296 (-67.1199, -24.2334) -> (-67.186, -24.22) construction
  line L1297 (-67.186, -24.22) -> (-67.2191, -24.2132) construction
  line L1298 (-5.6951, 60.7685) -> (-5.6979, 60.7993) construction
  line L1299 (-5.6979, 60.7993) -> (-5.7029, 60.8609) construction
  line L1300 (-5.7029, 60.8609) -> (-5.7078, 60.9533) construction
  line L1301 (-5.7078, 60.9533) -> (-5.7097, 61.0766) construction
  line L1302 (-5.7097, 61.0766) -> (-5.7056, 61.231) construction
  line L1303 (-5.7056, 61.231) -> (-5.6969, 61.3856) construction
  line L1304 (-5.6969, 61.3856) -> (-5.6854, 61.5403) construction
  line L1305 (-5.6854, 61.5403) -> (-5.6723, 61.695) construction
  line L1306 (-5.6723, 61.695) -> (-5.6583, 61.8498) construction
  line L1307 (-5.6583, 61.8498) -> (-5.6431, 62.0045) construction
  line L1308 (-5.6431, 62.0045) -> (-5.6265, 62.1593) construction
  line L1309 (-5.6265, 62.1593) -> (-5.608, 62.314) construction
  line L1310 (-5.608, 62.314) -> (-5.5871, 62.4688) construction
  line L1311 (-5.5871, 62.4688) -> (-5.5641, 62.6235) construction
  line L1312 (-5.5641, 62.6235) -> (-5.539, 62.7782) construction
  line L1313 (-5.539, 62.7782) -> (-5.5121, 62.9329) construction
  line L1314 (-5.5121, 62.9329) -> (-5.4838, 63.0875) construction
  line L1315 (-5.4838, 63.0875) -> (-5.4542, 63.2421) construction
  line L1316 (-5.4542, 63.2421) -> (-5.4233, 63.3966) construction
  line L1317 (-5.4233, 63.3966) -> (-5.3913, 63.5511) construction
  line L1318 (-5.3913, 63.5511) -> (-5.3579, 63.7055) construction
  line L1319 (-5.3579, 63.7055) -> (-5.3232, 63.8598) construction
  line L1320 (-5.3232, 63.8598) -> (-5.2871, 64.014) construction
  line L1321 (-5.2871, 64.014) -> (-5.2497, 64.1682) construction
  line L1322 (-5.2497, 64.1682) -> (-5.2109, 64.3222) construction
  line L1323 (-5.2109, 64.3222) -> (-5.1709, 64.4762) construction
  line L1324 (-5.1709, 64.4762) -> (-5.1297, 64.6301) construction
  line L1325 (-5.1297, 64.6301) -> (-5.0873, 64.7839) construction
  line L1326 (-5.0873, 64.7839) -> (-5.0439, 64.9376) construction
  line L1327 (-5.0439, 64.9376) -> (-4.9993, 65.0912) construction
  line L1328 (-4.9993, 65.0912) -> (-4.9536, 65.2447) construction
  line L1329 (-4.9536, 65.2447) -> (-4.9068, 65.398) construction
  line L1330 (-4.9068, 65.398) -> (-4.8589, 65.5513) construction
  line L1331 (-4.8589, 65.5513) -> (-4.8099, 65.7044) construction
  line L1332 (-4.8099, 65.7044) -> (-4.7599, 65.8574) construction
  line L1333 (-4.7599, 65.8574) -> (-4.7087, 66.0103) construction
  line L1334 (-4.7087, 66.0103) -> (-4.6566, 66.1631) construction
  line L1335 (-4.6566, 66.1631) -> (-4.6035, 66.3158) construction
  line L1336 (-4.6035, 66.3158) -> (-4.5493, 66.4683) construction
  line L1337 (-4.5493, 66.4683) -> (-4.4942, 66.6206) construction
  line L1338 (-4.4942, 66.6206) -> (-4.438, 66.7729) construction
  line L1339 (-4.438, 66.7729) -> (-4.381, 66.925) construction
  line L1340 (-4.381, 66.925) -> (-4.3229, 67.077) construction
  line L1341 (-4.3229, 67.077) -> (-4.2639, 67.2288) construction
  line L1342 (-4.2639, 67.2288) -> (-4.2039, 67.3804) construction
  line L1343 (-4.2039, 67.3804) -> (-4.143, 67.532) construction
  line L1344 (-4.143, 67.532) -> (-4.0812, 67.6833) construction
  line L1345 (-4.0812, 67.6833) -> (-4.0185, 67.8345) construction
  line L1346 (-4.0185, 67.8345) -> (-3.9548, 67.9856) construction
  line L1347 (-3.9548, 67.9856) -> (-3.8903, 68.1365) construction
  line L1348 (-3.8903, 68.1365) -> (-3.8249, 68.2872) construction
  line L1349 (-3.8249, 68.2872) -> (-3.7585, 68.4378) construction
  line L1350 (-3.7585, 68.4378) -> (-3.6913, 68.5882) construction
  line L1351 (-3.6913, 68.5882) -> (-3.6233, 68.7384) construction
  line L1352 (-3.6233, 68.7384) -> (-3.5543, 68.8885) construction
  line L1353 (-3.5543, 68.8885) -> (-3.4846, 69.0384) construction
  line L1354 (-3.4846, 69.0384) -> (-3.4139, 69.1881) construction
  line L1355 (-3.4139, 69.1881) -> (-3.3425, 69.3376) construction
  line L1356 (-3.3425, 69.3376) -> (-3.2701, 69.487) construction
  line L1357 (-3.2701, 69.487) -> (-3.197, 69.6362) construction
  line L1358 (-3.197, 69.6362) -> (-3.123, 69.7852) construction
  line L1359 (-3.123, 69.7852) -> (-3.0482, 69.934) construction
  line L1360 (-3.0482, 69.934) -> (-2.9726, 70.0826) construction
  line L1361 (-2.9726, 70.0826) -> (-2.8962, 70.2311) construction
  line L1362 (-2.8962, 70.2311) -> (-2.819, 70.3793) construction
  line L1363 (-2.819, 70.3793) -> (-2.741, 70.5274) construction
  line L1364 (-2.741, 70.5274) -> (-2.6622, 70.6752) construction
  line L1365 (-2.6622, 70.6752) -> (-2.5826, 70.8229) construction
  line L1366 (-2.5826, 70.8229) -> (-2.5023, 70.9703) construction
  line L1367 (-2.5023, 70.9703) -> (-2.4211, 71.1176) construction
  line L1368 (-2.4211, 71.1176) -> (-2.3556, 71.2352) construction
  line L1369 (-2.3556, 71.2352) -> (-2.3061, 71.3234) construction
  line L1370 (-2.3061, 71.3234) -> (-2.2729, 71.3821) construction
  line L1371 (-2.2729, 71.3821) -> (-2.2563, 71.4115) construction
  line L1372 (60.7685, 5.6951) -> (60.7993, 5.6979) construction
  line L1373 (60.7993, 5.6979) -> (60.8609, 5.7029) construction
  line L1374 (60.8609, 5.7029) -> (60.9533, 5.7078) construction
  line L1375 (60.9533, 5.7078) -> (61.0766, 5.7097) construction
  line L1376 (61.0766, 5.7097) -> (61.231, 5.7056) construction
  line L1377 (61.231, 5.7056) -> (61.3856, 5.6969) construction
  line L1378 (61.3856, 5.6969) -> (61.5403, 5.6854) construction
  line L1379 (61.5403, 5.6854) -> (61.695, 5.6723) construction
  line L1380 (61.695, 5.6723) -> (61.8498, 5.6583) construction
  line L1381 (61.8498, 5.6583) -> (62.0045, 5.6431) construction
  line L1382 (62.0045, 5.6431) -> (62.1593, 5.6265) construction
  line L1383 (62.1593, 5.6265) -> (62.314, 5.608) construction
  line L1384 (62.314, 5.608) -> (62.4688, 5.5871) construction
  line L1385 (62.4688, 5.5871) -> (62.6235, 5.5641) construction
  line L1386 (62.6235, 5.5641) -> (62.7782, 5.539) construction
  line L1387 (62.7782, 5.539) -> (62.9329, 5.5121) construction
  line L1388 (62.9329, 5.5121) -> (63.0875, 5.4838) construction
  line L1389 (63.0875, 5.4838) -> (63.2421, 5.4542) construction
  line L1390 (63.2421, 5.4542) -> (63.3966, 5.4233) construction
  line L1391 (63.3966, 5.4233) -> (63.5511, 5.3913) construction
  line L1392 (63.5511, 5.3913) -> (63.7055, 5.3579) construction
  line L1393 (63.7055, 5.3579) -> (63.8598, 5.3232) construction
  line L1394 (63.8598, 5.3232) -> (64.014, 5.2871) construction
  line L1395 (64.014, 5.2871) -> (64.1682, 5.2497) construction
  line L1396 (64.1682, 5.2497) -> (64.3222, 5.2109) construction
  line L1397 (64.3222, 5.2109) -> (64.4762, 5.1709) construction
  line L1398 (64.4762, 5.1709) -> (64.6301, 5.1297) construction
  line L1399 (64.6301, 5.1297) -> (64.7839, 5.0873) construction
  line L1400 (64.7839, 5.0873) -> (64.9376, 5.0439) construction
  line L1401 (64.9376, 5.0439) -> (65.0912, 4.9993) construction
  line L1402 (65.0912, 4.9993) -> (65.2447, 4.9536) construction
  line L1403 (65.2447, 4.9536) -> (65.398, 4.9068) construction
  line L1404 (65.398, 4.9068) -> (65.5513, 4.8589) construction
  line L1405 (65.5513, 4.8589) -> (65.7044, 4.8099) construction
  line L1406 (65.7044, 4.8099) -> (65.8574, 4.7599) construction
  line L1407 (65.8574, 4.7599) -> (66.0103, 4.7087) construction
  line L1408 (66.0103, 4.7087) -> (66.1631, 4.6566) construction
  line L1409 (66.1631, 4.6566) -> (66.3158, 4.6035) construction
  line L1410 (66.3158, 4.6035) -> (66.4683, 4.5493) construction
  line L1411 (66.4683, 4.5493) -> (66.6206, 4.4942) construction
  line L1412 (66.6206, 4.4942) -> (66.7729, 4.438) construction
  line L1413 (66.7729, 4.438) -> (66.925, 4.381) construction
  line L1414 (66.925, 4.381) -> (67.077, 4.3229) construction
  line L1415 (67.077, 4.3229) -> (67.2288, 4.2639) construction
  line L1416 (67.2288, 4.2639) -> (67.3804, 4.2039) construction
  line L1417 (67.3804, 4.2039) -> (67.532, 4.143) construction
  line L1418 (67.532, 4.143) -> (67.6833, 4.0812) construction
  line L1419 (67.6833, 4.0812) -> (67.8345, 4.0185) construction
  line L1420 (67.8345, 4.0185) -> (67.9856, 3.9548) construction
  line L1421 (67.9856, 3.9548) -> (68.1365, 3.8903) construction
  line L1422 (68.1365, 3.8903) -> (68.2872, 3.8249) construction
  line L1423 (68.2872, 3.8249) -> (68.4378, 3.7585) construction
  line L1424 (68.4378, 3.7585) -> (68.5882, 3.6913) construction
  line L1425 (68.5882, 3.6913) -> (68.7384, 3.6233) construction
  line L1426 (68.7384, 3.6233) -> (68.8885, 3.5543) construction
  line L1427 (68.8885, 3.5543) -> (69.0384, 3.4846) construction
  line L1428 (69.0384, 3.4846) -> (69.1881, 3.4139) construction
  line L1429 (69.1881, 3.4139) -> (69.3376, 3.3425) construction
  line L1430 (69.3376, 3.3425) -> (69.487, 3.2701) construction
  line L1431 (69.487, 3.2701) -> (69.6362, 3.197) construction
  line L1432 (69.6362, 3.197) -> (69.7852, 3.123) construction
  line L1433 (69.7852, 3.123) -> (69.934, 3.0482) construction
  line L1434 (69.934, 3.0482) -> (70.0826, 2.9726) construction
  line L1435 (70.0826, 2.9726) -> (70.2311, 2.8962) construction
  line L1436 (70.2311, 2.8962) -> (70.3793, 2.819) construction
  line L1437 (70.3793, 2.819) -> (70.5274, 2.741) construction
  line L1438 (70.5274, 2.741) -> (70.6752, 2.6622) construction
  line L1439 (70.6752, 2.6622) -> (70.8229, 2.5826) construction
  line L1440 (70.8229, 2.5826) -> (70.9703, 2.5023) construction
  line L1441 (70.9703, 2.5023) -> (71.1176, 2.4211) construction
  line L1442 (71.1176, 2.4211) -> (71.2352, 2.3556) construction
  line L1443 (71.2352, 2.3556) -> (71.3234, 2.3061) construction
  line L1444 (71.3234, 2.3061) -> (71.3821, 2.2729) construction
  line L1445 (71.3821, 2.2729) -> (71.4115, 2.2563) construction
  line L1446 (45.8153, 40.3263) -> (45.8385, 40.3467) construction
  line L1447 (45.8385, 40.3467) -> (45.8854, 40.3868) construction
  line L1448 (45.8854, 40.3868) -> (45.9573, 40.4451) construction
  line L1449 (45.9573, 40.4451) -> (46.056, 40.5192) construction
  line L1450 (46.056, 40.5192) -> (46.1833, 40.6066) construction
  line L1451 (46.1833, 40.6066) -> (46.3135, 40.6904) construction
  line L1452 (46.3135, 40.6904) -> (46.4454, 40.772) construction
  line L1453 (46.4454, 40.772) -> (46.5782, 40.8524) construction
  line L1454 (46.5782, 40.8524) -> (46.7117, 40.932) construction
  line L1455 (46.7117, 40.932) -> (46.8458, 41.0107) construction
  line L1456 (46.8458, 41.0107) -> (46.9807, 41.0883) construction
  line L1457 (46.9807, 41.0883) -> (47.1168, 41.1642) construction
  line L1458 (47.1168, 41.1642) -> (47.2543, 41.2383) construction
  line L1459 (47.2543, 41.2383) -> (47.393, 41.3106) construction
  line L1460 (47.393, 41.3106) -> (47.5329, 41.3813) construction
  line L1461 (47.5329, 41.3813) -> (47.6738, 41.4504) construction
  line L1462 (47.6738, 41.4504) -> (47.8156, 41.5184) construction
  line L1463 (47.8156, 41.5184) -> (47.9581, 41.5853) construction
  line L1464 (47.9581, 41.5853) -> (48.1012, 41.6512) construction
  line L1465 (48.1012, 41.6512) -> (48.245, 41.716) construction
  line L1466 (48.245, 41.716) -> (48.3895, 41.7798) construction
  line L1467 (48.3895, 41.7798) -> (48.5347, 41.8424) construction
  line L1468 (48.5347, 41.8424) -> (48.6807, 41.9039) construction
  line L1469 (48.6807, 41.9039) -> (48.8274, 41.9642) construction
  line L1470 (48.8274, 41.9642) -> (48.9749, 42.0234) construction
  line L1471 (48.9749, 42.0234) -> (49.123, 42.0815) construction
  line L1472 (49.123, 42.0815) -> (49.2717, 42.1386) construction
  line L1473 (49.2717, 42.1386) -> (49.421, 42.1947) construction
  line L1474 (49.421, 42.1947) -> (49.5709, 42.2499) construction
  line L1475 (49.5709, 42.2499) -> (49.7214, 42.3041) construction
  line L1476 (49.7214, 42.3041) -> (49.8724, 42.3574) construction
  line L1477 (49.8724, 42.3574) -> (50.024, 42.4097) construction
  line L1478 (50.024, 42.4097) -> (50.1761, 42.461) construction
  line L1479 (50.1761, 42.461) -> (50.3288, 42.5114) construction
  line L1480 (50.3288, 42.5114) -> (50.482, 42.5608) construction
  line L1481 (50.482, 42.5608) -> (50.6358, 42.6094) construction
  line L1482 (50.6358, 42.6094) -> (50.79, 42.657) construction
  line L1483 (50.79, 42.657) -> (50.9447, 42.7037) construction
  line L1484 (50.9447, 42.7037) -> (51.0999, 42.7495) construction
  line L1485 (51.0999, 42.7495) -> (51.2556, 42.7945) construction
  line L1486 (51.2556, 42.7945) -> (51.4118, 42.8386) construction